Autodesk Fusion 360 part; units mm, degrees
(part 2 of 2)
  spline S17 degree 5 poles (-46.9714, 7.0665) (-46.9528, 7.05) (-46.9154, 7.0172) (-46.8593, 6.9682) (-46.7843, 6.9032) (-46.6903, 6.8226) (-46.596, 6.7425) (-46.5014, 6.6629) (-46.4066, 6.584) (-46.3115, 6.5056) (-46.2162, 6.4278) (-46.1205, 6.3506) (-46.0246, 6.274) (-45.9285, 6.198) (-45.8321, 6.1226) (-45.7354, 6.0478) (-45.6384, 5.9737) (-45.5412, 5.9001) (-45.4438, 5.8272) (-45.3461, 5.7549) (-45.2481, 5.6832) (-45.1499, 5.6122) (-45.0514, 5.5418) (-44.9527, 5.4721) (-44.8537, 5.403) (-44.7544, 5.3346) (-44.6549, 5.2669) (-44.5552, 5.1998) (-44.4552, 5.1335) (-44.355, 5.0678) (-44.2545, 5.0028) (-44.1538, 4.9385) (-44.0528, 4.8749) (-43.9516, 4.8121) (-43.8501, 4.75) (-43.7484, 4.6886) (-43.6465, 4.6279) (-43.5443, 4.568) (-43.4418, 4.5089) (-43.3392, 4.4505) (-43.2363, 4.393) (-43.1331, 4.3362) (-43.0298, 4.2802) (-42.9261, 4.2251) (-42.8223, 4.1708) (-42.7182, 4.1174) (-42.6139, 4.0647) (-42.5093, 4.013) (-42.4045, 3.962) (-42.2995, 3.912) (-42.1943, 3.8629) (-42.0888, 3.8148) (-41.9831, 3.7677) (-41.8771, 3.7217) (-41.7709, 3.6767) (-41.6644, 3.6327) (-41.5578, 3.5897) (-41.4509, 3.5475) (-41.3439, 3.5063) (-41.2366, 3.4662) (-41.129, 3.4275) (-41.0212, 3.3903) (-40.913, 3.3548) (-40.8045, 3.321) (-40.6958, 3.2886) (-40.5869, 3.2574) (-40.4779, 3.2271) (-40.3687, 3.1975) (-40.2594, 3.1691) (-40.1498, 3.1428) (-40.0397, 3.1201) (-39.9511, 3.1058) (-39.8842, 3.0977) (-39.8395, 3.0936) (-39.8171, 3.0918) knots -1 -1 -1 -1 -1 -1 -0.98571429 -0.97142857 -0.95714286 -0.94285714 -0.92857143 -0.91428571 -0.9 -0.88571429 -0.87142857 -0.85714286 -0.84285714 -0.82857143 -0.81428571 -0.8 -0.78571429 -0.77142857 -0.75714286 -0.74285714 -0.72857143 -0.71428571 -0.7 -0.68571429 -0.67142857 -0.65714286 -0.64285714 -0.62857143 -0.61428571 -0.6 -0.58571429 -0.57142857 -0.55714286 -0.54285714 -0.52857143 -0.51428571 -0.5 -0.48571429 -0.47142857 -0.45714286 -0.44285714 -0.42857143 -0.41428571 -0.4 -0.38571429 -0.37142857 -0.35714286 -0.34285714 -0.32857143 -0.31428571 -0.3 -0.28571429 -0.27142857 -0.25714286 -0.24285714 -0.22857143 -0.21428571 -0.2 -0.18571429 -0.17142857 -0.15714286 -0.14285714 -0.12857143 -0.11428571 -0.1 -0.08571429 -0.07142857 -0.05714286 -0.04285714 -0.02857143 -0.01428571 0 0 0 0 0 0
  line L17 (-39.8171, 3.0918) -> (-37.889, 2.9415)
  arc A35 (-36.4259, 1.3021) -> (-37.889, 2.9415) centre (-38.0124, 1.3588) ccw
  arc A36 (-36.4259, 1.3021) -> (-36.4259, -1.3021) centre (0, 0) ccw
  arc A37 (-37.889, -2.9415) -> (-36.4259, -1.3021) centre (-38.0124, -1.3588) ccw
  line L18 (-37.889, -2.9415) -> (-39.8171, -3.0918)
  spline S18 degree 5 poles (-39.8171, -3.0918) (-39.8395, -3.0936) (-39.8842, -3.0977) (-39.9511, -3.1058) (-40.0397, -3.1201) (-40.1498, -3.1428) (-40.2594, -3.1691) (-40.3687, -3.1975) (-40.4779, -3.2271) (-40.5869, -3.2574) (-40.6958, -3.2886) (-40.8045, -3.321) (-40.913, -3.3548) (-41.0212, -3.3903) (-41.129, -3.4275) (-41.2366, -3.4662) (-41.3439, -3.5063) (-41.4509, -3.5475) (-41.5578, -3.5897) (-41.6644, -3.6327) (-41.7709, -3.6767) (-41.8771, -3.7217) (-41.9831, -3.7677) (-42.0888, -3.8148) (-42.1943, -3.8629) (-42.2995, -3.912) (-42.4045, -3.962) (-42.5093, -4.013) (-42.6139, -4.0647) (-42.7182, -4.1174) (-42.8223, -4.1708) (-42.9261, -4.2251) (-43.0298, -4.2802) (-43.1331, -4.3362) (-43.2363, -4.393) (-43.3392, -4.4505) (-43.4418, -4.5089) (-43.5443, -4.568) (-43.6465, -4.6279) (-43.7484, -4.6886) (-43.8501, -4.75) (-43.9516, -4.8121) (-44.0528, -4.8749) (-44.1538, -4.9385) (-44.2545, -5.0028) (-44.355, -5.0678) (-44.4552, -5.1335) (-44.5552, -5.1998) (-44.6549, -5.2669) (-44.7544, -5.3346) (-44.8537, -5.403) (-44.9527, -5.4721) (-45.0514, -5.5418) (-45.1499, -5.6122) (-45.2481, -5.6832) (-45.3461, -5.7549) (-45.4438, -5.8272) (-45.5412, -5.9001) (-45.6384, -5.9737) (-45.7354, -6.0478) (-45.8321, -6.1226) (-45.9285, -6.198) (-46.0246, -6.274) (-46.1205, -6.3506) (-46.2162, -6.4278) (-46.3115, -6.5056) (-46.4066, -6.584) (-46.5014, -6.6629) (-46.596, -6.7425) (-46.6903, -6.8226) (-46.7843, -6.9032) (-46.8593, -6.9682) (-46.9154, -7.0172) (-46.9528, -7.05) (-46.9714, -7.0665) knots 0 0 0 0 0 0 0.01428571 0.02857143 0.04285714 0.05714286 0.07142857 0.08571429 0.1 0.11428571 0.12857143 0.14285714 0.15714286 0.17142857 0.18571429 0.2 0.21428571 0.22857143 0.24285714 0.25714286 0.27142857 0.28571429 0.3 0.31428571 0.32857143 0.34285714 0.35714286 0.37142857 0.38571429 0.4 0.41428571 0.42857143 0.44285714 0.45714286 0.47142857 0.48571429 0.5 0.51428571 0.52857143 0.54285714 0.55714286 0.57142857 0.58571429 0.6 0.61428571 0.62857143 0.64285714 0.65714286 0.67142857 0.68571429 0.7 0.71428571 0.72857143 0.74285714 0.75714286 0.77142857 0.78571429 0.8 0.81428571 0.82857143 0.84285714 0.85714286 0.87142857 0.88571429 0.9 0.91428571 0.92857143 0.94285714 0.95714286 0.97142857 0.98571429 1 1 1 1 1 1
  arc A38 (-46.9714, -7.0665) -> (-46.3523, -10.3788) centre (0, 0) ccw
  spline S19 degree 5 poles (-46.3523, -10.3788) (-46.3289, -10.3873) (-46.2822, -10.4044) (-46.2122, -10.4298) (-46.1188, -10.4633) (-46.002, -10.5046) (-45.8851, -10.5453) (-45.7682, -10.5853) (-45.6513, -10.6246) (-45.5343, -10.6634) (-45.4173, -10.7015) (-45.3002, -10.7389) (-45.1831, -10.7757) (-45.066, -10.8118) (-44.9489, -10.8473) (-44.8317, -10.8821) (-44.7145, -10.9162) (-44.5973, -10.9497) (-44.4801, -10.9825) (-44.3629, -11.0146) (-44.2456, -11.0461) (-44.1284, -11.0768) (-44.0111, -11.1069) (-43.8939, -11.1362) (-43.7766, -11.1648) (-43.6594, -11.1928) (-43.5421, -11.22) (-43.4249, -11.2465) (-43.3077, -11.2723) (-43.1905, -11.2973) (-43.0733, -11.3216) (-42.9562, -11.3452) (-42.839, -11.368) (-42.7219, -11.39) (-42.6049, -11.4113) (-42.4879, -11.4318) (-42.3709, -11.4515) (-42.254, -11.4704) (-42.1371, -11.4886) (-42.0203, -11.5059) (-41.9036, -11.5224) (-41.7869, -11.5381) (-41.6703, -11.553) (-41.5537, -11.5669) (-41.4373, -11.58) (-41.3209, -11.5923) (-41.2046, -11.6037) (-41.0884, -11.6142) (-40.9723, -11.6238) (-40.8563, -11.6325) (-40.7404, -11.6403) (-40.6247, -11.647) (-40.5091, -11.6527) (-40.3937, -11.6573) (-40.2784, -11.6609) (-40.1632, -11.6635) (-40.0482, -11.6651) (-39.9333, -11.6659) (-39.8186, -11.6656) (-39.7041, -11.6642) (-39.5898, -11.6615) (-39.4758, -11.6572) (-39.3621, -11.6513) (-39.2488, -11.6436) (-39.1357, -11.6345) (-39.0229, -11.6242) (-38.9102, -11.6131) (-38.7978, -11.6013) (-38.6856, -11.5883) (-38.5739, -11.5732) (-38.463, -11.5546) (-38.3752, -11.536) (-38.31, -11.5193) (-38.2667, -11.507) (-38.2452, -11.5005) knots -1 -1 -1 -1 -1 -1 -0.98571429 -0.97142857 -0.95714286 -0.94285714 -0.92857143 -0.91428571 -0.9 -0.88571429 -0.87142857 -0.85714286 -0.84285714 -0.82857143 -0.81428571 -0.8 -0.78571429 -0.77142857 -0.75714286 -0.74285714 -0.72857143 -0.71428571 -0.7 -0.68571429 -0.67142857 -0.65714286 -0.64285714 -0.62857143 -0.61428571 -0.6 -0.58571429 -0.57142857 -0.55714286 -0.54285714 -0.52857143 -0.51428571 -0.5 -0.48571429 -0.47142857 -0.45714286 -0.44285714 -0.42857143 -0.41428571 -0.4 -0.38571429 -0.37142857 -0.35714286 -0.34285714 -0.32857143 -0.31428571 -0.3 -0.28571429 -0.27142857 -0.25714286 -0.24285714 -0.22857143 -0.21428571 -0.2 -0.18571429 -0.17142857 -0.15714286 -0.14285714 -0.12857143 -0.11428571 -0.1 -0.08571429 -0.07142857 -0.05714286 -0.04285714 -0.02857143 -0.01428571 0 0 0 0 0 0
  line L19 (-38.2452, -11.5005) -> (-36.3931, -10.9442)
  arc A39 (-34.4366, -11.9444) -> (-36.3931, -10.9442) centre (-35.9364, -12.4646) ccw
  arc A40 (-34.4366, -11.9444) -> (-33.4958, -14.3728) centre (0, 0) ccw
  arc A41 (-34.2679, -16.43) -> (-33.4958, -14.3728) centre (-34.9547, -14.9987) ccw
  line L20 (-34.2679, -16.43) -> (-36.0114, -17.2666)
  spline S20 degree 5 poles (-36.0114, -17.2666) (-36.0317, -17.2764) (-36.0719, -17.2964) (-36.1313, -17.328) (-36.2088, -17.3734) (-36.3032, -17.4344) (-36.3959, -17.4985) (-36.4876, -17.5644) (-36.5787, -17.6314) (-36.6694, -17.6991) (-36.7597, -17.7676) (-36.8494, -17.837) (-36.9384, -17.9077) (-37.0264, -17.9799) (-37.1135, -18.0535) (-37.1998, -18.1285) (-37.2854, -18.2046) (-37.3703, -18.2817) (-37.4547, -18.3597) (-37.5386, -18.4384) (-37.622, -18.5178) (-37.7048, -18.5982) (-37.787, -18.6794) (-37.8686, -18.7614) (-37.9496, -18.8444) (-38.03, -18.9282) (-38.1098, -19.0128) (-38.1891, -19.0981) (-38.2679, -19.1842) (-38.3462, -19.2709) (-38.4239, -19.3584) (-38.5012, -19.4465) (-38.5779, -19.5353) (-38.654, -19.6249) (-38.7297, -19.7151) (-38.8049, -19.8059) (-38.8795, -19.8974) (-38.9537, -19.9896) (-39.0273, -20.0823) (-39.1005, -20.1757) (-39.1731, -20.2697) (-39.2453, -20.3643) (-39.317, -20.4594) (-39.3882, -20.5552) (-39.4589, -20.6515) (-39.5291, -20.7484) (-39.5988, -20.8459) (-39.6681, -20.9439) (-39.7369, -21.0425) (-39.8052, -21.1416) (-39.873, -21.2412) (-39.9404, -21.3413) (-40.0072, -21.442) (-40.0737, -21.5432) (-40.1396, -21.6449) (-40.2051, -21.7472) (-40.2701, -21.8499) (-40.3346, -21.9531) (-40.3987, -22.0568) (-40.4623, -22.161) (-40.5254, -22.2656) (-40.5881, -22.3707) (-40.6503, -22.4764) (-40.712, -22.5824) (-40.7733, -22.6889) (-40.8341, -22.7959) (-40.8945, -22.9034) (-40.9544, -23.0112) (-41.0138, -23.1196) (-41.0728, -23.2283) (-41.1313, -23.3375) (-41.1778, -23.4252) (-41.2124, -23.4912) (-41.2354, -23.5353) (-41.2469, -23.5573) knots 0 0 0 0 0 0 0.01428571 0.02857143 0.04285714 0.05714286 0.07142857 0.08571429 0.1 0.11428571 0.12857143 0.14285714 0.15714286 0.17142857 0.18571429 0.2 0.21428571 0.22857143 0.24285714 0.25714286 0.27142857 0.28571429 0.3 0.31428571 0.32857143 0.34285714 0.35714286 0.37142857 0.38571429 0.4 0.41428571 0.42857143 0.44285714 0.45714286 0.47142857 0.48571429 0.5 0.51428571 0.52857143 0.54285714 0.55714286 0.57142857 0.58571429 0.6 0.61428571 0.62857143 0.64285714 0.65714286 0.67142857 0.68571429 0.7 0.71428571 0.72857143 0.74285714 0.75714286 0.77142857 0.78571429 0.8 0.81428571 0.82857143 0.84285714 0.85714286 0.87142857 0.88571429 0.9 0.91428571 0.92857143 0.94285714 0.95714286 0.97142857 0.98571429 1 1 1 1 1 1
  arc A42 (-41.2469, -23.5573) -> (-39.4729, -26.4223) centre (0, 0) ccw
  spline S21 degree 5 poles (-39.4729, -26.4223) (-39.4481, -26.4218) (-39.3984, -26.4209) (-39.3239, -26.4193) (-39.2247, -26.4168) (-39.1009, -26.4131) (-38.9772, -26.4088) (-38.8538, -26.4038) (-38.7305, -26.3983) (-38.6074, -26.3922) (-38.4845, -26.3854) (-38.3619, -26.378) (-38.2394, -26.3701) (-38.1171, -26.3614) (-37.9951, -26.3522) (-37.8732, -26.3423) (-37.7516, -26.3318) (-37.6303, -26.3207) (-37.5091, -26.309) (-37.3882, -26.2966) (-37.2675, -26.2835) (-37.1471, -26.2698) (-37.0269, -26.2555) (-36.9069, -26.2405) (-36.7873, -26.2248) (-36.6678, -26.2085) (-36.5487, -26.1916) (-36.4298, -26.1739) (-36.3112, -26.1556) (-36.1929, -26.1366) (-36.0748, -26.117) (-35.9571, -26.0966) (-35.8396, -26.0756) (-35.7225, -26.0538) (-35.6057, -26.0314) (-35.4891, -26.0082) (-35.3729, -25.9843) (-35.2571, -25.9598) (-35.1415, -25.9345) (-35.0264, -25.9084) (-34.9115, -25.8817) (-34.797, -25.8541) (-34.6829, -25.8258) (-34.5692, -25.7968) (-34.4559, -25.7669) (-34.343, -25.7363) (-34.2304, -25.7049) (-34.1183, -25.6727) (-34.0065, -25.6398) (-33.8952, -25.606) (-33.7844, -25.5714) (-33.674, -25.5359) (-33.5642, -25.4994) (-33.4549, -25.462) (-33.3461, -25.4237) (-33.2378, -25.3845) (-33.1299, -25.3445) (-33.0225, -25.3037) (-32.9157, -25.262) (-32.8094, -25.2193) (-32.7038, -25.1755) (-32.599, -25.1303) (-32.4951, -25.0837) (-32.3922, -25.0356) (-32.2901, -24.9863) (-32.1886, -24.9359) (-32.0876, -24.8849) (-31.987, -24.8332) (-31.8871, -24.7806) (-31.7884, -24.7261) (-31.6917, -24.6688) (-31.6165, -24.6197) (-31.5617, -24.5806) (-31.5259, -24.5535) (-31.5081, -24.5397) knots -1 -1 -1 -1 -1 -1 -0.98571429 -0.97142857 -0.95714286 -0.94285714 -0.92857143 -0.91428571 -0.9 -0.88571429 -0.87142857 -0.85714286 -0.84285714 -0.82857143 -0.81428571 -0.8 -0.78571429 -0.77142857 -0.75714286 -0.74285714 -0.72857143 -0.71428571 -0.7 -0.68571429 -0.67142857 -0.65714286 -0.64285714 -0.62857143 -0.61428571 -0.6 -0.58571429 -0.57142857 -0.55714286 -0.54285714 -0.52857143 -0.51428571 -0.5 -0.48571429 -0.47142857 -0.45714286 -0.44285714 -0.42857143 -0.41428571 -0.4 -0.38571429 -0.37142857 -0.35714286 -0.34285714 -0.32857143 -0.31428571 -0.3 -0.28571429 -0.27142857 -0.25714286 -0.24285714 -0.22857143 -0.21428571 -0.2 -0.18571429 -0.17142857 -0.15714286 -0.14285714 -0.12857143 -0.11428571 -0.1 -0.08571429 -0.07142857 -0.05714286 -0.04285714 -0.02857143 -0.01428571 0 0 0 0 0 0
  line L21 (-31.5081, -24.5397) -> (-29.982, -23.3519)
  arc A43 (-27.7963, -23.5777) -> (-29.982, -23.3519) centre (-29.007, -24.6046) ccw
  arc A44 (-27.7963, -23.5777) -> (-26.0419, -25.5023) centre (0, 0) ccw
  arc A45 (-26.0186, -27.6995) -> (-26.0419, -25.5023) centre (-27.1761, -26.613) ccw
  line L22 (-26.0186, -27.6995) -> (-27.3422, -29.1095)
  spline S22 degree 5 poles (-27.3422, -29.1095) (-27.3576, -29.1259) (-27.3879, -29.1591) (-27.4319, -29.21) (-27.4877, -29.2803) (-27.5537, -29.3713) (-27.617, -29.4646) (-27.6787, -29.5592) (-27.7394, -29.6546) (-27.7996, -29.7505) (-27.859, -29.8469) (-27.9176, -29.9441) (-27.975, -30.0421) (-28.031, -30.1412) (-28.0856, -30.2413) (-28.139, -30.3424) (-28.1913, -30.4444) (-28.2427, -30.5469) (-28.2932, -30.6501) (-28.343, -30.7538) (-28.392, -30.858) (-28.4402, -30.9628) (-28.4875, -31.0682) (-28.534, -31.1742) (-28.5795, -31.2808) (-28.6242, -31.388) (-28.6681, -31.4957) (-28.7113, -31.604) (-28.7536, -31.7127) (-28.7953, -31.8218) (-28.8362, -31.9315) (-28.8764, -32.0415) (-28.9158, -32.1521) (-28.9545, -32.2631) (-28.9925, -32.3745) (-29.0297, -32.4864) (-29.0663, -32.5987) (-29.1021, -32.7114) (-29.1373, -32.8245) (-29.1718, -32.938) (-29.2056, -33.0519) (-29.2387, -33.1662) (-29.2712, -33.2808) (-29.303, -33.3958) (-29.3341, -33.5112) (-29.3646, -33.6269) (-29.3944, -33.743) (-29.4236, -33.8594) (-29.4521, -33.9761) (-29.48, -34.0932) (-29.5073, -34.2106) (-29.5339, -34.3283) (-29.5599, -34.4464) (-29.5853, -34.5647) (-29.61, -34.6834) (-29.6341, -34.8024) (-29.6576, -34.9216) (-29.6805, -35.0412) (-29.7028, -35.161) (-29.7245, -35.2811) (-29.7455, -35.4015) (-29.766, -35.5222) (-29.7858, -35.6431) (-29.8051, -35.7644) (-29.8238, -35.8858) (-29.8418, -36.0076) (-29.8593, -36.1295) (-29.8762, -36.2518) (-29.8925, -36.3742) (-29.9082, -36.497) (-29.9233, -36.6199) (-29.9349, -36.7185) (-29.9434, -36.7925) (-29.9489, -36.8419) (-29.9517, -36.8666) knots 0 0 0 0 0 0 0.01428571 0.02857143 0.04285714 0.05714286 0.07142857 0.08571429 0.1 0.11428571 0.12857143 0.14285714 0.15714286 0.17142857 0.18571429 0.2 0.21428571 0.22857143 0.24285714 0.25714286 0.27142857 0.28571429 0.3 0.31428571 0.32857143 0.34285714 0.35714286 0.37142857 0.38571429 0.4 0.41428571 0.42857143 0.44285714 0.45714286 0.47142857 0.48571429 0.5 0.51428571 0.52857143 0.54285714 0.55714286 0.57142857 0.58571429 0.6 0.61428571 0.62857143 0.64285714 0.65714286 0.67142857 0.68571429 0.7 0.71428571 0.72857143 0.74285714 0.75714286 0.77142857 0.78571429 0.8 0.81428571 0.82857143 0.84285714 0.85714286 0.87142857 0.88571429 0.9 0.91428571 0.92857143 0.94285714 0.95714286 0.97142857 0.98571429 1 1 1 1 1 1
  arc A46 (-29.9517, -36.8666) -> (-27.2626, -38.8973) centre (0, 0) ccw
  spline S23 degree 5 poles (-27.2626, -38.8973) (-27.2396, -38.8879) (-27.1936, -38.8691) (-27.1247, -38.8407) (-27.0331, -38.8025) (-26.9189, -38.7543) (-26.8052, -38.7056) (-26.6919, -38.6565) (-26.5789, -38.6068) (-26.4664, -38.5566) (-26.3542, -38.5059) (-26.2425, -38.4547) (-26.1312, -38.403) (-26.0203, -38.3508) (-25.9098, -38.2981) (-25.7998, -38.2449) (-25.6902, -38.1912) (-25.581, -38.137) (-25.4723, -38.0822) (-25.364, -38.027) (-25.2562, -37.9712) (-25.1489, -37.9149) (-25.042, -37.8582) (-24.9355, -37.8009) (-24.8296, -37.743) (-24.7241, -37.6847) (-24.6191, -37.6258) (-24.5147, -37.5664) (-24.4107, -37.5065) (-24.3072, -37.4461) (-24.2042, -37.3851) (-24.1018, -37.3236) (-23.9999, -37.2615) (-23.8985, -37.1989) (-23.7977, -37.1358) (-23.6974, -37.0721) (-23.5977, -37.0079) (-23.4985, -36.9431) (-23.3999, -36.8778) (-23.3019, -36.8119) (-23.2045, -36.7454) (-23.1077, -36.6784) (-23.0115, -36.6108) (-22.916, -36.5426) (-22.8211, -36.4738) (-22.7268, -36.4045) (-22.6332, -36.3346) (-22.5403, -36.2641) (-22.448, -36.193) (-22.3564, -36.1213) (-22.2655, -36.0489) (-22.1755, -35.9759) (-22.0862, -35.9023) (-21.9978, -35.8279) (-21.9102, -35.7529) (-21.8233, -35.6772) (-21.7372, -35.601) (-21.6519, -35.5241) (-21.5673, -35.4466) (-21.4835, -35.3684) (-21.4009, -35.2894) (-21.3195, -35.2095) (-21.2395, -35.1285) (-21.1609, -35.0464) (-21.0835, -34.9635) (-21.0071, -34.8799) (-20.9313, -34.7959) (-20.8562, -34.7113) (-20.782, -34.6261) (-20.7097, -34.5397) (-20.6402, -34.4513) (-20.5879, -34.3784) (-20.5509, -34.3221) (-20.5272, -34.2839) (-20.5157, -34.2646) knots -1 -1 -1 -1 -1 -1 -0.98571429 -0.97142857 -0.95714286 -0.94285714 -0.92857143 -0.91428571 -0.9 -0.88571429 -0.87142857 -0.85714286 -0.84285714 -0.82857143 -0.81428571 -0.8 -0.78571429 -0.77142857 -0.75714286 -0.74285714 -0.72857143 -0.71428571 -0.7 -0.68571429 -0.67142857 -0.65714286 -0.64285714 -0.62857143 -0.61428571 -0.6 -0.58571429 -0.57142857 -0.55714286 -0.54285714 -0.52857143 -0.51428571 -0.5 -0.48571429 -0.47142857 -0.45714286 -0.44285714 -0.42857143 -0.41428571 -0.4 -0.38571429 -0.37142857 -0.35714286 -0.34285714 -0.32857143 -0.31428571 -0.3 -0.28571429 -0.27142857 -0.25714286 -0.24285714 -0.22857143 -0.21428571 -0.2 -0.18571429 -0.17142857 -0.15714286 -0.14285714 -0.12857143 -0.11428571 -0.1 -0.08571429 -0.07142857 -0.05714286 -0.04285714 -0.02857143 -0.01428571 0 0 0 0 0 0
  line L23 (-20.5157, -34.2646) -> (-19.5217, -32.6057)
  arc A47 (-17.402, -32.0268) -> (-19.5217, -32.6057) centre (-18.16, -33.4216) ccw
  arc A48 (-17.402, -32.0268) -> (-15.0708, -33.1876) centre (0, 0) ccw
  arc A49 (-14.2554, -35.228) -> (-15.0708, -33.1876) centre (-15.7272, -34.633) ccw
  line L24 (-14.2554, -35.228) -> (-14.9803, -37.0209)
  spline S24 degree 5 poles (-14.9803, -37.0209) (-14.9887, -37.0418) (-15.005, -37.0837) (-15.0276, -37.1471) (-15.0542, -37.2328) (-15.0829, -37.3415) (-15.1083, -37.4513) (-15.1316, -37.5618) (-15.1538, -37.6727) (-15.1752, -37.7839) (-15.1958, -37.8953) (-15.2153, -38.007) (-15.2334, -38.1192) (-15.2499, -38.2318) (-15.2646, -38.3449) (-15.2779, -38.4585) (-15.2898, -38.5724) (-15.3007, -38.6866) (-15.3106, -38.8011) (-15.3195, -38.9157) (-15.3276, -39.0306) (-15.3347, -39.1458) (-15.3407, -39.2611) (-15.3457, -39.3768) (-15.3497, -39.4926) (-15.3526, -39.6087) (-15.3547, -39.725) (-15.3558, -39.8415) (-15.356, -39.9582) (-15.3554, -40.075) (-15.354, -40.192) (-15.3517, -40.3092) (-15.3485, -40.4265) (-15.3445, -40.544) (-15.3397, -40.6616) (-15.334, -40.7794) (-15.3275, -40.8973) (-15.3202, -41.0154) (-15.3121, -41.1336) (-15.3033, -41.2518) (-15.2937, -41.3702) (-15.2833, -41.4888) (-15.2722, -41.6074) (-15.2603, -41.7261) (-15.2476, -41.8449) (-15.2342, -41.9638) (-15.2201, -42.0829) (-15.2053, -42.2019) (-15.1897, -42.3211) (-15.1734, -42.4404) (-15.1564, -42.5597) (-15.1387, -42.6791) (-15.1203, -42.7986) (-15.1012, -42.9181) (-15.0814, -43.0377) (-15.0609, -43.1573) (-15.0398, -43.277) (-15.0179, -43.3968) (-14.9954, -43.5165) (-14.9722, -43.6364) (-14.9484, -43.7563) (-14.9239, -43.8762) (-14.8987, -43.9961) (-14.8729, -44.1161) (-14.8464, -44.2361) (-14.8192, -44.3562) (-14.7915, -44.4762) (-14.7631, -44.5963) (-14.734, -44.7164) (-14.7043, -44.8365) (-14.674, -44.9566) (-14.6493, -45.0527) (-14.6304, -45.1248) (-14.6177, -45.1729) (-14.6113, -45.1969) knots 0 0 0 0 0 0 0.01428571 0.02857143 0.04285714 0.05714286 0.07142857 0.08571429 0.1 0.11428571 0.12857143 0.14285714 0.15714286 0.17142857 0.18571429 0.2 0.21428571 0.22857143 0.24285714 0.25714286 0.27142857 0.28571429 0.3 0.31428571 0.32857143 0.34285714 0.35714286 0.37142857 0.38571429 0.4 0.41428571 0.42857143 0.44285714 0.45714286 0.47142857 0.48571429 0.5 0.51428571 0.52857143 0.54285714 0.55714286 0.57142857 0.58571429 0.6 0.61428571 0.62857143 0.64285714 0.65714286 0.67142857 0.68571429 0.7 0.71428571 0.72857143 0.74285714 0.75714286 0.77142857 0.78571429 0.8 0.81428571 0.82857143 0.84285714 0.85714286 0.87142857 0.88571429 0.9 0.91428571 0.92857143 0.94285714 0.95714286 0.97142857 0.98571429 1 1 1 1 1 1
  arc A50 (-14.6113, -45.1969) -> (-11.3703, -46.119) centre (0, 0) ccw
  spline S25 degree 5 poles (-11.3703, -46.119) (-11.3522, -46.102) (-11.3161, -46.0678) (-11.2621, -46.0164) (-11.1905, -45.9478) (-11.1015, -45.8616) (-11.013, -45.7751) (-10.9251, -45.6883) (-10.8377, -45.6011) (-10.7509, -45.5137) (-10.6647, -45.4259) (-10.579, -45.3378) (-10.4939, -45.2494) (-10.4093, -45.1607) (-10.3253, -45.0716) (-10.242, -44.9823) (-10.1592, -44.8926) (-10.0769, -44.8026) (-9.9953, -44.7123) (-9.9143, -44.6216) (-9.8339, -44.5307) (-9.7542, -44.4395) (-9.675, -44.3479) (-9.5965, -44.256) (-9.5186, -44.1638) (-9.4413, -44.0713) (-9.3647, -43.9785) (-9.2887, -43.8854) (-9.2134, -43.7919) (-9.1387, -43.6982) (-9.0647, -43.6041) (-8.9914, -43.5097) (-8.9188, -43.4151) (-8.8469, -43.3201) (-8.7757, -43.2248) (-8.7052, -43.1292) (-8.6354, -43.0333) (-8.5663, -42.937) (-8.498, -42.8405) (-8.4304, -42.7437) (-8.3636, -42.6465) (-8.2975, -42.5491) (-8.2323, -42.4513) (-8.1678, -42.3532) (-8.1042, -42.2548) (-8.0413, -42.1561) (-7.9793, -42.057) (-7.9181, -41.9577) (-7.8577, -41.8581) (-7.7982, -41.7581) (-7.7396, -41.6579) (-7.682, -41.5573) (-7.6254, -41.4563) (-7.5698, -41.3551) (-7.5152, -41.2534) (-7.4616, -41.1515) (-7.4088, -41.0493) (-7.357, -40.9468) (-7.3061, -40.844) (-7.2562, -40.7408) (-7.2077, -40.6373) (-7.1607, -40.5333) (-7.1154, -40.4289) (-7.0718, -40.324) (-7.0295, -40.2188) (-6.9884, -40.1132) (-6.9481, -40.0074) (-6.9086, -39.9015) (-6.8703, -39.7952) (-6.834, -39.6885) (-6.8012, -39.581) (-6.7787, -39.4941) (-6.7645, -39.4283) (-6.7563, -39.3841) (-6.7525, -39.3619) knots -1 -1 -1 -1 -1 -1 -0.98571429 -0.97142857 -0.95714286 -0.94285714 -0.92857143 -0.91428571 -0.9 -0.88571429 -0.87142857 -0.85714286 -0.84285714 -0.82857143 -0.81428571 -0.8 -0.78571429 -0.77142857 -0.75714286 -0.74285714 -0.72857143 -0.71428571 -0.7 -0.68571429 -0.67142857 -0.65714286 -0.64285714 -0.62857143 -0.61428571 -0.6 -0.58571429 -0.57142857 -0.55714286 -0.54285714 -0.52857143 -0.51428571 -0.5 -0.48571429 -0.47142857 -0.45714286 -0.44285714 -0.42857143 -0.41428571 -0.4 -0.38571429 -0.37142857 -0.35714286 -0.34285714 -0.32857143 -0.31428571 -0.3 -0.28571429 -0.27142857 -0.25714286 -0.24285714 -0.22857143 -0.21428571 -0.2 -0.18571429 -0.17142857 -0.15714286 -0.14285714 -0.12857143 -0.11428571 -0.1 -0.08571429 -0.07142857 -0.05714286 -0.04285714 -0.02857143 -0.01428571 0 0 0 0 0 0
  line L25 (-6.7525, -39.3619) -> (-6.4249, -37.456)
  arc A51 (-4.6575, -36.1504) -> (-6.4249, -37.456) centre (-4.8604, -37.7249) ccw
  arc A52 (-4.6575, -36.1504) -> (-2.0644, -36.3907) centre (0, 0) ccw
  arc A53 (-0.567, -37.9988) -> (-2.0644, -36.3907) centre (-2.1543, -37.9756) ccw
  line L26 (-0.567, -37.9988) -> (-0.5952, -39.9325)
  spline S26 degree 5 poles (-0.5952, -39.9325) (-0.5955, -39.955) (-0.5956, -39.9999) (-0.5937, -40.0672) (-0.5876, -40.1568) (-0.5751, -40.2685) (-0.5591, -40.3801) (-0.5409, -40.4915) (-0.5215, -40.6029) (-0.5013, -40.7143) (-0.4803, -40.8256) (-0.4582, -40.9369) (-0.4345, -41.048) (-0.4092, -41.159) (-0.3821, -41.2698) (-0.3534, -41.3805) (-0.3234, -41.491) (-0.2922, -41.6014) (-0.2601, -41.7117) (-0.2271, -41.8219) (-0.1931, -41.9319) (-0.1581, -42.0418) (-0.122, -42.1516) (-0.0849, -42.2612) (-0.0468, -42.3707) (-0.0076, -42.48) (0.0325, -42.5892) (0.0736, -42.6983) (0.1155, -42.8071) (0.1583, -42.9159) (0.2019, -43.0244) (0.2464, -43.1329) (0.2917, -43.2411) (0.3379, -43.3492) (0.3849, -43.4572) (0.4327, -43.565) (0.4814, -43.6726) (0.5308, -43.78) (0.581, -43.8873) (0.632, -43.9944) (0.6837, -44.1013) (0.7362, -44.2081) (0.7895, -44.3147) (0.8434, -44.4211) (0.8981, -44.5273) (0.9536, -44.6334) (1.0097, -44.7392) (1.0666, -44.8449) (1.1242, -44.9504) (1.1824, -45.0557) (1.2414, -45.1609) (1.301, -45.2658) (1.3614, -45.3706) (1.4223, -45.4751) (1.484, -45.5795) (1.5463, -45.6836) (1.6093, -45.7876) (1.6729, -45.8914) (1.7372, -45.9949) (1.8021, -46.0983) (1.8676, -46.2015) (1.9338, -46.3044) (2.0006, -46.4072) (2.0681, -46.5097) (2.1361, -46.6121) (2.2048, -46.7142) (2.274, -46.8161) (2.3439, -46.9178) (2.4144, -47.0193) (2.4854, -47.1206) (2.5571, -47.2217) (2.6149, -47.3023) (2.6585, -47.3627) (2.6877, -47.403) (2.7023, -47.4231) knots 0 0 0 0 0 0 0.01428571 0.02857143 0.04285714 0.05714286 0.07142857 0.08571429 0.1 0.11428571 0.12857143 0.14285714 0.15714286 0.17142857 0.18571429 0.2 0.21428571 0.22857143 0.24285714 0.25714286 0.27142857 0.28571429 0.3 0.31428571 0.32857143 0.34285714 0.35714286 0.37142857 0.38571429 0.4 0.41428571 0.42857143 0.44285714 0.45714286 0.47142857 0.48571429 0.5 0.51428571 0.52857143 0.54285714 0.55714286 0.57142857 0.58571429 0.6 0.61428571 0.62857143 0.64285714 0.65714286 0.67142857 0.68571429 0.7 0.71428571 0.72857143 0.74285714 0.75714286 0.77142857 0.78571429 0.8 0.81428571 0.82857143 0.84285714 0.85714286 0.87142857 0.88571429 0.9 0.91428571 0.92857143 0.94285714 0.95714286 0.97142857 0.98571429 1 1 1 1 1 1
  arc A54 (2.7023, -47.4231) -> (6.0576, -47.1122) centre (0, 0) ccw
  spline S27 degree 5 poles (6.0576, -47.1122) (6.0683, -47.0897) (6.0896, -47.0448) (6.1214, -46.9774) (6.1634, -46.8875) (6.2153, -46.775) (6.2665, -46.6624) (6.3171, -46.5497) (6.3671, -46.4368) (6.4165, -46.3239) (6.4652, -46.2109) (6.5133, -46.0978) (6.5607, -45.9846) (6.6075, -45.8714) (6.6537, -45.758) (6.6991, -45.6445) (6.7439, -45.531) (6.7881, -45.4174) (6.8316, -45.3037) (6.8744, -45.1899) (6.9165, -45.0761) (6.9579, -44.9622) (6.9986, -44.8482) (7.0387, -44.7341) (7.078, -44.62) (7.1167, -44.5059) (7.1546, -44.3916) (7.1918, -44.2773) (7.2283, -44.163) (7.264, -44.0486) (7.299, -43.9342) (7.3333, -43.8197) (7.3668, -43.7052) (7.3995, -43.5906) (7.4315, -43.476) (7.4627, -43.3614) (7.4932, -43.2468) (7.5228, -43.1321) (7.5516, -43.0174) (7.5797, -42.9027) (7.6069, -42.788) (7.6333, -42.6732) (7.6588, -42.5585) (7.6835, -42.4437) (7.7073, -42.329) (7.7302, -42.2142) (7.7523, -42.0995) (7.7735, -41.9848) (7.7938, -41.87) (7.8132, -41.7553) (7.8316, -41.6407) (7.849, -41.5261) (7.8653, -41.4115) (7.8806, -41.297) (7.8948, -41.1825) (7.9079, -41.0681) (7.9202, -40.9537) (7.9315, -40.8394) (7.9418, -40.7251) (7.951, -40.611) (7.9589, -40.4969) (7.9651, -40.383) (7.9697, -40.2692) (7.9725, -40.1557) (7.9738, -40.0423) (7.974, -39.929) (7.9734, -39.8158) (7.972, -39.7027) (7.9694, -39.5898) (7.9646, -39.4772) (7.9564, -39.3651) (7.9459, -39.2759) (7.9354, -39.2094) (7.9271, -39.1652) (7.9227, -39.1432) knots -1 -1 -1 -1 -1 -1 -0.98571429 -0.97142857 -0.95714286 -0.94285714 -0.92857143 -0.91428571 -0.9 -0.88571429 -0.87142857 -0.85714286 -0.84285714 -0.82857143 -0.81428571 -0.8 -0.78571429 -0.77142857 -0.75714286 -0.74285714 -0.72857143 -0.71428571 -0.7 -0.68571429 -0.67142857 -0.65714286 -0.64285714 -0.62857143 -0.61428571 -0.6 -0.58571429 -0.57142857 -0.55714286 -0.54285714 -0.52857143 -0.51428571 -0.5 -0.48571429 -0.47142857 -0.45714286 -0.44285714 -0.42857143 -0.41428571 -0.4 -0.38571429 -0.37142857 -0.35714286 -0.34285714 -0.32857143 -0.31428571 -0.3 -0.28571429 -0.27142857 -0.25714286 -0.24285714 -0.22857143 -0.21428571 -0.2 -0.18571429 -0.17142857 -0.15714286 -0.14285714 -0.12857143 -0.11428571 -0.1 -0.08571429 -0.07142857 -0.05714286 -0.04285714 -0.02857143 -0.01428571 0 0 0 0 0 0
  line L27 (7.9227, -39.1432) -> (7.5396, -37.2476)
  arc A55 (8.716, -35.3917) -> (7.5396, -37.2476) centre (9.0956, -36.9332) ccw
  arc A56 (8.716, -35.3917) -> (11.2208, -34.6791) centre (0, 0) ccw
  arc A57 (13.1981, -35.6377) -> (11.2208, -34.6791) centre (11.7095, -36.1895) ccw
  line L28 (13.1981, -35.6377) -> (13.8703, -37.451)
  spline S28 degree 5 poles (13.8703, -37.451) (13.8781, -37.472) (13.8943, -37.5139) (13.9203, -37.576) (13.9584, -37.6574) (14.0104, -37.757) (14.0656, -37.8552) (14.1229, -37.9526) (14.1812, -38.0495) (14.2402, -38.1461) (14.3, -38.2423) (14.3609, -38.338) (14.4231, -38.4331) (14.4868, -38.5274) (14.5521, -38.621) (14.6188, -38.7138) (14.6867, -38.806) (14.7557, -38.8977) (14.8255, -38.989) (14.8961, -39.0798) (14.9675, -39.1701) (15.0399, -39.26) (15.1131, -39.3493) (15.1873, -39.4381) (15.2625, -39.5264) (15.3385, -39.6142) (15.4153, -39.7015) (15.493, -39.7884) (15.5714, -39.8747) (15.6506, -39.9607) (15.7305, -40.0462) (15.8111, -40.1312) (15.8925, -40.2158) (15.9746, -40.2999) (16.0574, -40.3836) (16.141, -40.4668) (16.2252, -40.5496) (16.3101, -40.6319) (16.3957, -40.7138) (16.4819, -40.7952) (16.5688, -40.8763) (16.6563, -40.9569) (16.7444, -41.037) (16.8332, -41.1167) (16.9226, -41.196) (17.0126, -41.2749) (17.1032, -41.3533) (17.1944, -41.4313) (17.2862, -41.5089) (17.3786, -41.5861) (17.4716, -41.6628) (17.5651, -41.7391) (17.6592, -41.815) (17.7538, -41.8905) (17.849, -41.9655) (17.9447, -42.0401) (18.041, -42.1143) (18.1378, -42.1881) (18.2352, -42.2615) (18.333, -42.3344) (18.4314, -42.4069) (18.5303, -42.479) (18.6297, -42.5507) (18.7297, -42.622) (18.8301, -42.6928) (18.931, -42.7633) (19.0324, -42.8333) (19.1343, -42.9029) (19.2367, -42.972) (19.3395, -43.0408) (19.4428, -43.1092) (19.5259, -43.1635) (19.5884, -43.2041) (19.6301, -43.231) (19.651, -43.2445) knots 0 0 0 0 0 0 0.01428571 0.02857143 0.04285714 0.05714286 0.07142857 0.08571429 0.1 0.11428571 0.12857143 0.14285714 0.15714286 0.17142857 0.18571429 0.2 0.21428571 0.22857143 0.24285714 0.25714286 0.27142857 0.28571429 0.3 0.31428571 0.32857143 0.34285714 0.35714286 0.37142857 0.38571429 0.4 0.41428571 0.42857143 0.44285714 0.45714286 0.47142857 0.48571429 0.5 0.51428571 0.52857143 0.54285714 0.55714286 0.57142857 0.58571429 0.6 0.61428571 0.62857143 0.64285714 0.65714286 0.67142857 0.68571429 0.7 0.71428571 0.72857143 0.74285714 0.75714286 0.77142857 0.78571429 0.8 0.81428571 0.82857143 0.84285714 0.85714286 0.87142857 0.88571429 0.9 0.91428571 0.92857143 0.94285714 0.95714286 0.97142857 0.98571429 1 1 1 1 1 1
  arc A58 (19.651, -43.2445) -> (22.6675, -41.7425) centre (0, 0) ccw
  spline S29 degree 5 poles (22.6675, -41.7425) (22.6693, -41.7177) (22.673, -41.6681) (22.6782, -41.5938) (22.6849, -41.4948) (22.6926, -41.3711) (22.6998, -41.2476) (22.7062, -41.1242) (22.7121, -41.001) (22.7173, -40.8779) (22.722, -40.7549) (22.7259, -40.6321) (22.7293, -40.5094) (22.732, -40.3869) (22.734, -40.2645) (22.7355, -40.1423) (22.7362, -40.0202) (22.7364, -39.8983) (22.7358, -39.7766) (22.7346, -39.655) (22.7328, -39.5337) (22.7303, -39.4125) (22.7271, -39.2915) (22.7232, -39.1707) (22.7187, -39.0501) (22.7135, -38.9296) (22.7075, -38.8094) (22.701, -38.6894) (22.6937, -38.5696) (22.6857, -38.4501) (22.677, -38.3307) (22.6676, -38.2116) (22.6575, -38.0927) (22.6466, -37.974) (22.635, -37.8556) (22.6227, -37.7375) (22.6097, -37.6196) (22.5959, -37.5019) (22.5814, -37.3846) (22.5661, -37.2675) (22.55, -37.1506) (22.5332, -37.0341) (22.5155, -36.9179) (22.4971, -36.802) (22.4778, -36.6864) (22.4577, -36.5711) (22.4369, -36.4562) (22.4152, -36.3415) (22.3927, -36.2272) (22.3693, -36.1133) (22.3451, -35.9997) (22.3199, -35.8865) (22.2937, -35.7738) (22.2666, -35.6615) (22.2385, -35.5496) (22.2094, -35.4382) (22.1795, -35.3271) (22.1488, -35.2164) (22.1172, -35.1061) (22.0845, -34.9963) (22.0506, -34.8872) (22.0153, -34.7787) (21.9784, -34.671) (21.94, -34.564) (21.9003, -34.4578) (21.8596, -34.3521) (21.8181, -34.2468) (21.7759, -34.1418) (21.7327, -34.0375) (21.6876, -33.9342) (21.6394, -33.8326) (21.5975, -33.7533) (21.5636, -33.6951) (21.5399, -33.6569) (21.5278, -33.638) knots -1 -1 -1 -1 -1 -1 -0.98571429 -0.97142857 -0.95714286 -0.94285714 -0.92857143 -0.91428571 -0.9 -0.88571429 -0.87142857 -0.85714286 -0.84285714 -0.82857143 -0.81428571 -0.8 -0.78571429 -0.77142857 -0.75714286 -0.74285714 -0.72857143 -0.71428571 -0.7 -0.68571429 -0.67142857 -0.65714286 -0.64285714 -0.62857143 -0.61428571 -0.6 -0.58571429 -0.57142857 -0.55714286 -0.54285714 -0.52857143 -0.51428571 -0.5 -0.48571429 -0.47142857 -0.45714286 -0.44285714 -0.42857143 -0.41428571 -0.4 -0.38571429 -0.37142857 -0.35714286 -0.34285714 -0.32857143 -0.31428571 -0.3 -0.28571429 -0.27142857 -0.25714286 -0.24285714 -0.22857143 -0.21428571 -0.2 -0.18571429 -0.17142857 -0.15714286 -0.14285714 -0.12857143 -0.11428571 -0.1 -0.08571429 -0.07142857 -0.05714286 -0.04285714 -0.02857143 -0.01428571 0 0 0 0 0 0
  line L29 (21.5278, -33.638) -> (20.4859, -32.0088)
  arc A59 (20.9124, -29.8532) -> (20.4859, -32.0088) centre (21.8232, -31.1534) ccw
  arc A60 (20.9124, -29.8532) -> (22.9906, -28.2838) centre (0, 0) ccw
  arc A61 (25.1806, -28.4634) -> (22.9906, -28.2838) centre (23.992, -29.5157) ccw
  line L30 (25.1806, -28.4634) -> (26.4625, -29.9115)
  spline S30 degree 5 poles (26.4625, -29.9115) (26.4774, -29.9283) (26.5076, -29.9615) (26.5544, -30.01) (26.6192, -30.0721) (26.7037, -30.1462) (26.7907, -30.2179) (26.8792, -30.288) (26.9686, -30.3573) (27.0586, -30.426) (27.1491, -30.4941) (27.2404, -30.5614) (27.3327, -30.6276) (27.4262, -30.6925) (27.5209, -30.7561) (27.6167, -30.8186) (27.7133, -30.8801) (27.8107, -30.9407) (27.9088, -31.0006) (28.0074, -31.0597) (28.1067, -31.1181) (28.2066, -31.1758) (28.3072, -31.2326) (28.4085, -31.2887) (28.5104, -31.3438) (28.613, -31.3983) (28.7162, -31.4519) (28.82, -31.5048) (28.9243, -31.5571) (29.0292, -31.6086) (29.1346, -31.6594) (29.2405, -31.7096) (29.3469, -31.7591) (29.4539, -31.8079) (29.5613, -31.856) (29.6693, -31.9034) (29.7777, -31.9501) (29.8867, -31.9962) (29.996, -32.0417) (30.1059, -32.0865) (30.2161, -32.1307) (30.3269, -32.1742) (30.438, -32.2171) (30.5496, -32.2594) (30.6616, -32.301) (30.774, -32.342) (30.8868, -32.3824) (31.0001, -32.4222) (31.1137, -32.4614) (31.2277, -32.5) (31.3421, -32.538) (31.4569, -32.5753) (31.572, -32.6121) (31.6875, -32.6483) (31.8034, -32.6839) (31.9196, -32.7189) (32.0362, -32.7533) (32.1531, -32.7871) (32.2704, -32.8203) (32.388, -32.853) (32.5059, -32.8851) (32.6242, -32.9166) (32.7428, -32.9475) (32.8617, -32.9779) (32.981, -33.0077) (33.1005, -33.0369) (33.2203, -33.0655) (33.3405, -33.0936) (33.4609, -33.1212) (33.5817, -33.1481) (33.7027, -33.1745) (33.7998, -33.1952) (33.8727, -33.2105) (33.9214, -33.2205) (33.9458, -33.2255) knots 0 0 0 0 0 0 0.01428571 0.02857143 0.04285714 0.05714286 0.07142857 0.08571429 0.1 0.11428571 0.12857143 0.14285714 0.15714286 0.17142857 0.18571429 0.2 0.21428571 0.22857143 0.24285714 0.25714286 0.27142857 0.28571429 0.3 0.31428571 0.32857143 0.34285714 0.35714286 0.37142857 0.38571429 0.4 0.41428571 0.42857143 0.44285714 0.45714286 0.47142857 0.48571429 0.5 0.51428571 0.52857143 0.54285714 0.55714286 0.57142857 0.58571429 0.6 0.61428571 0.62857143 0.64285714 0.65714286 0.67142857 0.68571429 0.7 0.71428571 0.72857143 0.74285714 0.75714286 0.77142857 0.78571429 0.8 0.81428571 0.82857143 0.84285714 0.85714286 0.87142857 0.88571429 0.9 0.91428571 0.92857143 0.94285714 0.95714286 0.97142857 0.98571429 1 1 1 1 1 1
  arc A62 (33.9458, -33.2255) -> (36.2159, -30.7353) centre (0, 0) ccw
  spline S31 degree 5 poles (36.2159, -30.7353) (36.2087, -30.7115) (36.1942, -30.664) (36.1723, -30.5927) (36.1427, -30.498) (36.1052, -30.3799) (36.0673, -30.2622) (36.0287, -30.1448) (35.9897, -30.0277) (35.9501, -29.911) (35.91, -29.7947) (35.8693, -29.6787) (35.8281, -29.5631) (35.7864, -29.4479) (35.7441, -29.333) (35.7012, -29.2185) (35.6579, -29.1044) (35.6139, -28.9907) (35.5695, -28.8774) (35.5245, -28.7645) (35.4789, -28.652) (35.4328, -28.5399) (35.3861, -28.4283) (35.3388, -28.317) (35.291, -28.2062) (35.2427, -28.0958) (35.1937, -27.9858) (35.1442, -27.8763) (35.0942, -27.7672) (35.0435, -27.6586) (34.9923, -27.5504) (34.9405, -27.4428) (34.8881, -27.3356) (34.8351, -27.2288) (34.7816, -27.1226) (34.7274, -27.0169) (34.6727, -26.9116) (34.6173, -26.8069) (34.5614, -26.7027) (34.5048, -26.5991) (34.4476, -26.4959) (34.3898, -26.3934) (34.3314, -26.2914) (34.2723, -26.19) (34.2126, -26.0891) (34.1522, -25.9889) (34.0912, -25.8892) (34.0296, -25.7902) (33.9673, -25.6917) (33.9044, -25.5939) (33.8407, -25.4967) (33.7764, -25.4003) (33.7113, -25.3046) (33.6454, -25.2097) (33.5788, -25.1156) (33.5114, -25.0221) (33.4434, -24.9293) (33.3748, -24.8372) (33.3054, -24.7458) (33.2353, -24.6553) (33.1643, -24.5657) (33.0921, -24.4773) (33.0189, -24.3902) (32.9445, -24.3044) (32.869, -24.2196) (32.7929, -24.1358) (32.7161, -24.0526) (32.6389, -23.97) (32.5609, -23.8883) (32.4815, -23.8082) (32.3999, -23.7309) (32.3321, -23.6721) (32.2795, -23.6301) (32.2437, -23.603) (32.2255, -23.5897) knots -1 -1 -1 -1 -1 -1 -0.98571429 -0.97142857 -0.95714286 -0.94285714 -0.92857143 -0.91428571 -0.9 -0.88571429 -0.87142857 -0.85714286 -0.84285714 -0.82857143 -0.81428571 -0.8 -0.78571429 -0.77142857 -0.75714286 -0.74285714 -0.72857143 -0.71428571 -0.7 -0.68571429 -0.67142857 -0.65714286 -0.64285714 -0.62857143 -0.61428571 -0.6 -0.58571429 -0.57142857 -0.55714286 -0.54285714 -0.52857143 -0.51428571 -0.5 -0.48571429 -0.47142857 -0.45714286 -0.44285714 -0.42857143 -0.41428571 -0.4 -0.38571429 -0.37142857 -0.35714286 -0.34285714 -0.32857143 -0.31428571 -0.3 -0.28571429 -0.27142857 -0.25714286 -0.24285714 -0.22857143 -0.21428571 -0.2 -0.18571429 -0.17142857 -0.15714286 -0.14285714 -0.12857143 -0.11428571 -0.1 -0.08571429 -0.07142857 -0.05714286 -0.04285714 -0.02857143 -0.01428571 0 0 0 0 0 0
  line L31 (32.2255, -23.5897) -> (30.6654, -22.4469)
  arc A63 (30.2845, -20.2829) -> (30.6654, -22.4469) centre (31.6035, -21.1663) ccw
  arc A64 (30.2845, -20.2829) -> (31.6554, -18.0687) centre (0, 0) ccw
  arc A65 (33.7624, -17.4451) -> (31.6554, -18.0687) centre (33.0341, -18.8557) ccw
  line L32 (33.7624, -17.4451) -> (35.4808, -18.3323)
  spline S32 degree 5 poles (35.4808, -18.3323) (35.5008, -18.3426) (35.541, -18.3626) (35.6021, -18.391) (35.6849, -18.4254) (35.7905, -18.464) (35.8975, -18.4994) (36.0054, -18.5328) (36.1138, -18.5651) (36.2225, -18.5967) (36.3315, -18.6275) (36.441, -18.6573) (36.551, -18.6856) (36.6616, -18.7124) (36.7729, -18.7375) (36.8848, -18.7612) (36.9971, -18.7836) (37.1098, -18.805) (37.2229, -18.8254) (37.3362, -18.8449) (37.4499, -18.8635) (37.5639, -18.8812) (37.6782, -18.8978) (37.7929, -18.9135) (37.9079, -18.9281) (38.0232, -18.9418) (38.1388, -18.9545) (38.2547, -18.9664) (38.3709, -18.9774) (38.4873, -18.9876) (38.6039, -18.9969) (38.7208, -19.0054) (38.8379, -19.0131) (38.9552, -19.02) (39.0728, -19.026) (39.1906, -19.0312) (39.3086, -19.0356) (39.4269, -19.0393) (39.5453, -19.0422) (39.6639, -19.0443) (39.7826, -19.0456) (39.9016, -19.0462) (40.0208, -19.0461) (40.1401, -19.0452) (40.2596, -19.0435) (40.3792, -19.0412) (40.499, -19.0381) (40.619, -19.0343) (40.7391, -19.0298) (40.8593, -19.0246) (40.9797, -19.0187) (41.1002, -19.0121) (41.2209, -19.0048) (41.3416, -18.9968) (41.4625, -18.9881) (41.5836, -18.9787) (41.7047, -18.9687) (41.826, -18.958) (41.9473, -18.9466) (42.0688, -18.9346) (42.1903, -18.9219) (42.312, -18.9086) (42.4338, -18.8946) (42.5556, -18.8799) (42.6776, -18.8646) (42.7996, -18.8487) (42.9217, -18.8321) (43.0439, -18.8149) (43.1661, -18.7971) (43.2885, -18.7786) (43.4109, -18.7595) (43.5089, -18.7437) (43.5824, -18.7316) (43.6314, -18.7234) (43.6559, -18.7193) knots 0 0 0 0 0 0 0.01428571 0.02857143 0.04285714 0.05714286 0.07142857 0.08571429 0.1 0.11428571 0.12857143 0.14285714 0.15714286 0.17142857 0.18571429 0.2 0.21428571 0.22857143 0.24285714 0.25714286 0.27142857 0.28571429 0.3 0.31428571 0.32857143 0.34285714 0.35714286 0.37142857 0.38571429 0.4 0.41428571 0.42857143 0.44285714 0.45714286 0.47142857 0.48571429 0.5 0.51428571 0.52857143 0.54285714 0.55714286 0.57142857 0.58571429 0.6 0.61428571 0.62857143 0.64285714 0.65714286 0.67142857 0.68571429 0.7 0.71428571 0.72857143 0.74285714 0.75714286 0.77142857 0.78571429 0.8 0.81428571 0.82857143 0.84285714 0.85714286 0.87142857 0.88571429 0.9 0.91428571 0.92857143 0.94285714 0.95714286 0.97142857 0.98571429 1 1 1 1 1 1
  arc A66 (43.6559, -18.7193) -> (44.8732, -15.5771) centre (0, 0) ccw
  spline S33 degree 5 poles (44.8732, -15.5771) (44.8579, -15.5575) (44.8272, -15.5184) (44.781, -15.46) (44.7192, -15.3823) (44.6416, -15.2857) (44.5637, -15.1896) (44.4853, -15.0941) (44.4066, -14.9991) (44.3276, -14.9045) (44.2481, -14.8106) (44.1683, -14.7171) (44.0881, -14.6242) (44.0076, -14.5318) (43.9267, -14.44) (43.8454, -14.3487) (43.7637, -14.258) (43.6817, -14.1678) (43.5993, -14.0782) (43.5165, -13.9892) (43.4334, -13.9008) (43.3499, -13.8129) (43.266, -13.7256) (43.1818, -13.6389) (43.0972, -13.5529) (43.0122, -13.4674) (42.9268, -13.3825) (42.8411, -13.2983) (42.755, -13.2147) (42.6686, -13.1317) (42.5817, -13.0493) (42.4945, -12.9676) (42.4069, -12.8866) (42.319, -12.8062) (42.2307, -12.7265) (42.142, -12.6475) (42.0529, -12.5692) (41.9635, -12.4915) (41.8737, -12.4145) (41.7835, -12.3383) (41.6929, -12.2628) (41.6019, -12.188) (41.5106, -12.114) (41.4189, -12.0408) (41.3268, -11.9684) (41.2343, -11.8967) (41.1414, -11.8258) (41.0481, -11.7557) (40.9545, -11.6864) (40.8605, -11.6179) (40.766, -11.5503) (40.6712, -11.4837) (40.5759, -11.418) (40.4802, -11.3533) (40.384, -11.2895) (40.2875, -11.2267) (40.1906, -11.1648) (40.0933, -11.1037) (39.9956, -11.0435) (39.8975, -10.9844) (39.7989, -10.9265) (39.6997, -10.8701) (39.5999, -10.8154) (39.4995, -10.7622) (39.3986, -10.7105) (39.2973, -10.6598) (39.1957, -10.6099) (39.0938, -10.5608) (38.9916, -10.5128) (38.8887, -10.4668) (38.7846, -10.4242) (38.7001, -10.3939) (38.6359, -10.3737) (38.5927, -10.3614) (38.571, -10.3556) knots -1 -1 -1 -1 -1 -1 -0.98571429 -0.97142857 -0.95714286 -0.94285714 -0.92857143 -0.91428571 -0.9 -0.88571429 -0.87142857 -0.85714286 -0.84285714 -0.82857143 -0.81428571 -0.8 -0.78571429 -0.77142857 -0.75714286 -0.74285714 -0.72857143 -0.71428571 -0.7 -0.68571429 -0.67142857 -0.65714286 -0.64285714 -0.62857143 -0.61428571 -0.6 -0.58571429 -0.57142857 -0.55714286 -0.54285714 -0.52857143 -0.51428571 -0.5 -0.48571429 -0.47142857 -0.45714286 -0.44285714 -0.42857143 -0.41428571 -0.4 -0.38571429 -0.37142857 -0.35714286 -0.34285714 -0.32857143 -0.31428571 -0.3 -0.28571429 -0.27142857 -0.25714286 -0.24285714 -0.22857143 -0.21428571 -0.2 -0.18571429 -0.17142857 -0.15714286 -0.14285714 -0.12857143 -0.11428571 -0.1 -0.08571429 -0.07142857 -0.05714286 -0.04285714 -0.02857143 -0.01428571 0 0 0 0 0 0
  line L33 (38.571, -10.3556) -> (36.7034, -9.8535)
  arc A67 (35.5664, -7.9732) -> (36.7034, -9.8535) centre (37.1155, -8.3205) ccw
  circle A68 centre (0, 0) radius 10
  circle A69 centre (0, 0) radius 10
  circle A70 centre (0, 0) radius 22.5
  dimension "d8" = 45
  constraint concentric A0 A69
  constraint concentric A0 A70
  measures "d8" diameter of A70
extrude "Extrude3" add sketch "Sketch1 (2)" along normal blind 50 contours A70 in component "Spur Gear (17 teeth)"
sketch "Sketch2 (2)" plane through (0, 0, 0) normal (0, 1, 0) x (1, 0, 0)
  line L0 (-29.9517, -20) -> (-27.2626, -20)
  line L1 (-29.9517, -20) -> (-29.9517, -70)
  circle A0 centre (0, -45) radius 10
  point P0 (-29.9517, -20)
  dimension "d11" = 50
  constraint coincident P0 L0.start
  constraint perpendicular L0 L1
  measures "d11" distance of P0 L1.end
extrude "Extrude4" cut sketch "Sketch2 (2)" along normal blind 25 in component "Spur Gear (17 teeth)"
thread "Thread1" "ISO Metric profile 14.0 M14x2 6H" major diameter 14.2505 minor diameter 12.0225 pitch 2 angle 60 resizes the face on face at (-9.9585, 7.4338, 45.9103) in component "Spur Gear (17 teeth)"
fillet "Fillet2" radius 1 4 edges at (-20.9774, -8.1363, 70) (-9.3233, 3.6162, 70) (-20.9774, 8.1363, 20) (-9.3233, 3.6162, 0) in component "Spur Gear (17 teeth)"
component "Spur Gear (17 teeth)" placed x (1, 0, 0) y (0, 1, 0) z (0, 0, 1) at (0, 0, 0)
